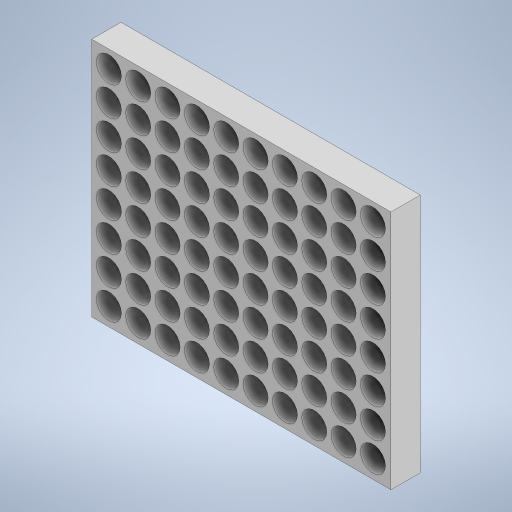
# Autodesk Inventor part: FullCellGrid
Saved by Autodesk Inventor 2024 (Build 280153000, 153)
## iProperties
Created: 2024-10-23
Part Number: FullCellGrid
Material: Generic
Document SubType Name: Modeling
Designer: v
Density: 1 g/cm^3
Appearance: Default
Author: v
Autodesk Inventor part; units mm, degrees
ref_plane "YZ Plane" through (0, 0, 0) normal (1, 0, 0) x (0, 1, 0)
ref_plane "XZ Plane" through (0, 0, 0) normal (0, 1, 0) x (-1, 0, 0)
ref_plane "XY Plane" through (0, 0, 0) normal (0, 0, 1) x (1, 0, 0)
sketch "Sketch1" plane through (0, 0, 0) normal (0, 0, 1) x (1, 0, 0)
  line L0 (-136.7692, 87.9231) -> (122.3108, 87.9231)
  line L1 (122.3108, 87.9231) -> (122.3108, -120.3569)
  line L2 (122.3108, -120.3569) -> (-136.7692, -120.3569)
  line L3 (-136.7692, -120.3569) -> (-136.7692, 87.9231)
  circle A0 centre (-121.8594, 73.0133) radius 10.8585
  circle A1 centre (-121.8594, 47.6133) radius 10.8585
  circle A2 centre (-121.8594, 22.2133) radius 10.8585
  circle A3 centre (-121.8594, -3.1867) radius 10.8585
  circle A4 centre (-121.8594, -28.5867) radius 10.8585
  circle A5 centre (-121.8594, -53.9867) radius 10.8585
  circle A6 centre (-121.8594, -79.3867) radius 10.8585
  circle A7 centre (-121.8594, -104.7867) radius 10.8585
  circle A8 centre (-96.4594, 73.0133) radius 10.8585
  circle A9 centre (-96.4594, 47.6133) radius 10.8585
  circle A10 centre (-96.4594, 22.2133) radius 10.8585
  circle A11 centre (-96.4594, -3.1867) radius 10.8585
  circle A12 centre (-96.4594, -28.5867) radius 10.8585
  circle A13 centre (-96.4594, -53.9867) radius 10.8585
  circle A14 centre (-96.4594, -79.3867) radius 10.8585
  circle A15 centre (-96.4594, -104.7867) radius 10.8585
  circle A16 centre (-71.0594, 73.0133) radius 10.8585
  circle A17 centre (-71.0594, 47.6133) radius 10.8585
  circle A18 centre (-71.0594, 22.2133) radius 10.8585
  circle A19 centre (-71.0594, -3.1867) radius 10.8585
  circle A20 centre (-71.0594, -28.5867) radius 10.8585
  circle A21 centre (-71.0594, -53.9867) radius 10.8585
  circle A22 centre (-71.0594, -79.3867) radius 10.8585
  circle A23 centre (-71.0594, -104.7867) radius 10.8585
  circle A24 centre (-45.6594, 73.0133) radius 10.8585
  circle A25 centre (-45.6594, 47.6133) radius 10.8585
  circle A26 centre (-45.6594, 22.2133) radius 10.8585
  circle A27 centre (-45.6594, -3.1867) radius 10.8585
  circle A28 centre (-45.6594, -28.5867) radius 10.8585
  circle A29 centre (-45.6594, -53.9867) radius 10.8585
  circle A30 centre (-45.6594, -79.3867) radius 10.8585
  circle A31 centre (-45.6594, -104.7867) radius 10.8585
  circle A32 centre (-20.2594, 73.0133) radius 10.8585
  circle A33 centre (-20.2594, 47.6133) radius 10.8585
  circle A34 centre (-20.2594, 22.2133) radius 10.8585
  circle A35 centre (-20.2594, -3.1867) radius 10.8585
  circle A36 centre (-20.2594, -28.5867) radius 10.8585
  circle A37 centre (-20.2594, -53.9867) radius 10.8585
  circle A38 centre (-20.2594, -79.3867) radius 10.8585
  circle A39 centre (-20.2594, -104.7867) radius 10.8585
  circle A40 centre (5.1406, 73.0133) radius 10.8585
  circle A41 centre (5.1406, 47.6133) radius 10.8585
  circle A42 centre (5.1406, 22.2133) radius 10.8585
  circle A43 centre (5.1406, -3.1867) radius 10.8585
  circle A44 centre (5.1406, -28.5867) radius 10.8585
  circle A45 centre (5.1406, -53.9867) radius 10.8585
  circle A46 centre (5.1406, -79.3867) radius 10.8585
  circle A47 centre (5.1406, -104.7867) radius 10.8585
  circle A48 centre (30.5406, 73.0133) radius 10.8585
  circle A49 centre (30.5406, 47.6133) radius 10.8585
  circle A50 centre (30.5406, 22.2133) radius 10.8585
  circle A51 centre (30.5406, -3.1867) radius 10.8585
  circle A52 centre (30.5406, -28.5867) radius 10.8585
  circle A53 centre (30.5406, -53.9867) radius 10.8585
  circle A54 centre (30.5406, -79.3867) radius 10.8585
  circle A55 centre (30.5406, -104.7867) radius 10.8585
  circle A56 centre (55.9406, 73.0133) radius 10.8585
  circle A57 centre (55.9406, 47.6133) radius 10.8585
  circle A58 centre (55.9406, 22.2133) radius 10.8585
  circle A59 centre (55.9406, -3.1867) radius 10.8585
  circle A60 centre (55.9406, -28.5867) radius 10.8585
  circle A61 centre (55.9406, -53.9867) radius 10.8585
  circle A62 centre (55.9406, -79.3867) radius 10.8585
  circle A63 centre (55.9406, -104.7867) radius 10.8585
  circle A64 centre (81.3406, 73.0133) radius 10.8585
  circle A65 centre (81.3406, 47.6133) radius 10.8585
  circle A66 centre (81.3406, 22.2133) radius 10.8585
  circle A67 centre (81.3406, -3.1867) radius 10.8585
  circle A68 centre (81.3406, -28.5867) radius 10.8585
  circle A69 centre (81.3406, -53.9867) radius 10.8585
  circle A70 centre (81.3406, -79.3867) radius 10.8585
  circle A71 centre (81.3406, -104.7867) radius 10.8585
  circle A72 centre (106.7406, 73.0133) radius 10.8585
  circle A73 centre (106.7406, 47.6133) radius 10.8585
  circle A74 centre (106.7406, 22.2133) radius 10.8585
  circle A75 centre (106.7406, -3.1867) radius 10.8585
  circle A76 centre (106.7406, -28.5867) radius 10.8585
  circle A77 centre (106.7406, -53.9867) radius 10.8585
  circle A78 centre (106.7406, -79.3867) radius 10.8585
  circle A79 centre (106.7406, -104.7867) radius 10.8585
  dimension "d0" = 259.08
  dimension "d6" = 25.4
  dimension "d9" = 25.4
  dimension "d12" = 208.28
  dimension "d28" = 21.717
  constraints: 80 centre point, 8 end point, 2 horizontal, 2 parallel, 1 perpendicular, 1 vertical, 158 other
  measures "d0" distance of L0.start L0.end
  measures "d6" distance of A0.centre A1.centre
  measures "d9" distance of A0.centre A8.centre
  measures "d12" distance of L2.end L0.start
  measures "d28" diameter of A0
extrude "Extrusion1" add sketch "Sketch1" against normal blind 25.4 contours L0 L1 L2 L3 | A0 | A1 | A2 | A3 | A4 | A5 | A6 | A7 | A8 | A9 | A10 | A11 | A12 | A13 | A14 | A15 | A16 | A17 | A18 | A19 | A20 | A21 | A22 | A23 | A24 | A25 | A26 | A27 | A28 | A29 | A30 | A31 | A32 | A33 | A34 | A35 | A36 | A37 | A38 | A39 | A40 | A41 | A42 | A43 | A44 | A45 | A46 | A47 | A48 | A49 | A50 | A51 | A52 | A53 | A54 | A55 | A56 | A57 | A58 | A59 | A60 | A61 | A62 | A63 | A64 | A65 | A66 | A67 | A68 | A69 | A70 | A71 | A72 | A73 | A74 | A75 | A76 | A77 | A78 | A79
sketch "Sketch2" plane through (0, 0, 0) normal (0, 0, 1) x (1, 0, 0)
  line L0 (-136.7692, -120.3569) -> (122.3108, -120.3569) projected
  line L1 (122.3108, -120.3569) -> (122.3108, 87.9231) projected
  line L2 (122.3108, 87.9231) -> (-136.7692, 87.9231) projected
  line L3 (-136.7692, 87.9231) -> (-136.7692, -120.3569) projected
  circle A0 centre (-121.8594, 73.0133) radius 10.8585
  circle A1 centre (-121.8594, 47.6133) radius 10.8585
  circle A2 centre (-121.8594, 22.2133) radius 10.8585
  circle A3 centre (-121.8594, -3.1867) radius 10.8585
  circle A4 centre (-121.8594, -28.5867) radius 10.8585
  circle A5 centre (-121.8594, -53.9867) radius 10.8585
  circle A6 centre (-121.8594, -79.3867) radius 10.8585
  circle A7 centre (-121.8594, -104.7867) radius 10.8585
  circle A8 centre (-96.4594, 73.0133) radius 10.8585
  circle A9 centre (-96.4594, 47.6133) radius 10.8585
  circle A10 centre (-96.4594, 22.2133) radius 10.8585
  circle A11 centre (-96.4594, -3.1867) radius 10.8585
  circle A12 centre (-96.4594, -28.5867) radius 10.8585
  circle A13 centre (-96.4594, -53.9867) radius 10.8585
  circle A14 centre (-96.4594, -79.3867) radius 10.8585
  circle A15 centre (-96.4594, -104.7867) radius 10.8585
  circle A16 centre (-71.0594, 73.0133) radius 10.8585
  circle A17 centre (-71.0594, 47.6133) radius 10.8585
  circle A18 centre (-71.0594, 22.2133) radius 10.8585
  circle A19 centre (-71.0594, -3.1867) radius 10.8585
  circle A20 centre (-71.0594, -28.5867) radius 10.8585
  circle A21 centre (-71.0594, -53.9867) radius 10.8585
  circle A22 centre (-71.0594, -79.3867) radius 10.8585
  circle A23 centre (-71.0594, -104.7867) radius 10.8585
  circle A24 centre (-45.6594, 73.0133) radius 10.8585
  circle A25 centre (-45.6594, 47.6133) radius 10.8585
  circle A26 centre (-45.6594, 22.2133) radius 10.8585
  circle A27 centre (-45.6594, -3.1867) radius 10.8585
  circle A28 centre (-45.6594, -28.5867) radius 10.8585
  circle A29 centre (-45.6594, -53.9867) radius 10.8585
  circle A30 centre (-45.6594, -79.3867) radius 10.8585
  circle A31 centre (-45.6594, -104.7867) radius 10.8585
  circle A32 centre (-20.2594, 73.0133) radius 10.8585
  circle A33 centre (-20.2594, 47.6133) radius 10.8585
  circle A34 centre (-20.2594, 22.2133) radius 10.8585
  circle A35 centre (-20.2594, -3.1867) radius 10.8585
  circle A36 centre (-20.2594, -28.5867) radius 10.8585
  circle A37 centre (-20.2594, -53.9867) radius 10.8585
  circle A38 centre (-20.2594, -79.3867) radius 10.8585
  circle A39 centre (-20.2594, -104.7867) radius 10.8585
  circle A40 centre (5.1406, 73.0133) radius 10.8585
  circle A41 centre (5.1406, 47.6133) radius 10.8585
  circle A42 centre (5.1406, 22.2133) radius 10.8585
  circle A43 centre (5.1406, -3.1867) radius 10.8585
  circle A44 centre (5.1406, -28.5867) radius 10.8585
  circle A45 centre (5.1406, -53.9867) radius 10.8585
  circle A46 centre (5.1406, -79.3867) radius 10.8585
  circle A47 centre (5.1406, -104.7867) radius 10.8585
  circle A48 centre (30.5406, 73.0133) radius 10.8585
  circle A49 centre (30.5406, 47.6133) radius 10.8585
  circle A50 centre (30.5406, 22.2133) radius 10.8585
  circle A51 centre (30.5406, -3.1867) radius 10.8585
  circle A52 centre (30.5406, -28.5867) radius 10.8585
  circle A53 centre (30.5406, -53.9867) radius 10.8585
  circle A54 centre (30.5406, -79.3867) radius 10.8585
  circle A55 centre (30.5406, -104.7867) radius 10.8585
  circle A56 centre (55.9406, 73.0133) radius 10.8585
  circle A57 centre (55.9406, 47.6133) radius 10.8585
  circle A58 centre (55.9406, 22.2133) radius 10.8585
  circle A59 centre (55.9406, -3.1867) radius 10.8585
  circle A60 centre (55.9406, -28.5867) radius 10.8585
  circle A61 centre (55.9406, -53.9867) radius 10.8585
  circle A62 centre (55.9406, -79.3867) radius 10.8585
  circle A63 centre (55.9406, -104.7867) radius 10.8585
  circle A64 centre (81.3406, 73.0133) radius 10.8585
  circle A65 centre (81.3406, 47.6133) radius 10.8585
  circle A66 centre (81.3406, 22.2133) radius 10.8585
  circle A67 centre (81.3406, -3.1867) radius 10.8585
  circle A68 centre (81.3406, -28.5867) radius 10.8585
  circle A69 centre (81.3406, -53.9867) radius 10.8585
  circle A70 centre (81.3406, -79.3867) radius 10.8585
  circle A71 centre (81.3406, -104.7867) radius 10.8585
  circle A72 centre (106.7406, 73.0133) radius 10.8585
  circle A73 centre (106.7406, 47.6133) radius 10.8585
  circle A74 centre (106.7406, 22.2133) radius 10.8585
  circle A75 centre (106.7406, -3.1867) radius 10.8585
  circle A76 centre (106.7406, -28.5867) radius 10.8585
  circle A77 centre (106.7406, -53.9867) radius 10.8585
  circle A78 centre (106.7406, -79.3867) radius 10.8585
  circle A79 centre (106.7406, -104.7867) radius 10.8585
  point P0 (0, 0)
  dimension "d15" = 14.9098
  dimension "d16" = 14.9098
  dimension "d17" = 21.717
  dimension "d20" = 25.4
  dimension "d23" = 25.4
  constraints: 80 centre point, 1 horizontal, 1 vertical, 158 other
  measures "d15" distance from line of L2 A0.centre
  measures "d16" distance from line of L3 A0.centre
  measures "d17" diameter of A0
  measures "d20" distance of A0.centre A1.centre
  measures "d23" distance of A0.centre A8.centre
extrude "Extrusion2" cut sketch "Sketch2" against normal through all contours A0 | A1 | A2 | A3 | A4 | A5 | A6 | A7 | A8 | A9 | A10 | A11 | A12 | A13 | A14 | A15 | A16 | A17 | A18 | A19 | A20 | A21 | A22 | A23 | A24 | A25 | A26 | A27 | A28 | A29 | A30 | A31 | A32 | A33 | A34 | A35 | A36 | A37 | A38 | A39 | A40 | A41 | A42 | A43 | A44 | A45 | A46 | A47 | A48 | A49 | A50 | A51 | A52 | A53 | A54 | A55 | A56 | A57 | A58 | A59 | A60 | A61 | A62 | A63 | A64 | A65 | A66 | A67 | A68 | A69 | A70 | A71 | A72 | A73 | A74 | A75 | A76 | A77 | A78 | A79
body "Solid1"
